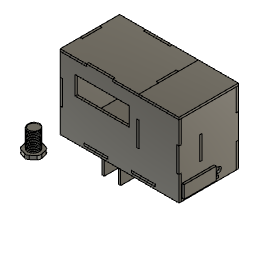
Tetrabytes (Autodesk Fusion 360 design; units mm, degrees)
Autodesk Fusion 360 part; units mm, degrees
note: some values were not read from the file. Chosen so that the rebuilt part matches the saved one: which face or edge a step refers to; which bodies a step acts on; where a thread starts. Set by a fixed rule: which sketch regions a step uses.
(part 1 of 2)
sketch "Sketch1" plane through (0, 0, 0) normal (0, 1, 0) x (1, 0, 0) in component "Front"
  line L0 (0, 0) -> (160, 0)
  line L1 (160, 0) -> (160, -100)
  line L2 (160, -100) -> (0, -100)
  line L3 (0, -100) -> (0, 0)
  line L4 (3, 0) -> (3, -100) construction
  line L5 (0, -3) -> (160, -3) construction
  line L6 (160, -6) -> (0, -6) construction
  line L7 (32, -3) -> (64, -3)
  line L8 (64, -3) -> (64, -6)
  line L9 (64, -6) -> (32, -6)
  line L10 (32, -6) -> (32, -3)
  line L11 (96, -3) -> (128, -3)
  line L12 (128, -3) -> (128, -6)
  line L13 (128, -6) -> (96, -6)
  line L14 (96, -6) -> (96, -3)
  line L15 (0, -66.6667) -> (3, -66.6667)
  line L16 (3, -66.6667) -> (3, -33.3333)
  line L17 (3, -33.3333) -> (0, -33.3333)
  line L18 (0, -33.3333) -> (0, -66.6667)
  line L19 (80, -100) -> (80, -87.8783) construction
  line L20 (157, -66.6667) -> (157, -33.3333)
  line L21 (160, -66.6667) -> (157, -66.6667)
  line L22 (157, -33.3333) -> (160, -33.3333)
  line L23 (160, -33.3333) -> (160, -66.6667)
  line L24 (157, 0) -> (157, -100) construction
  dimension "d1" = 160
  dimension "d8" = 100
  dimension "d9" = 3
  dimension "d10" = 3
  dimension "d11" = 3
  dimension "d12" = 32
  dimension "d13" = 32
  dimension "d14" = 32
  dimension "d15" = 32
  dimension "d16" = 33.3333
  dimension "d17" = 33.3333
  constraint horizontal L0
  constraint vertical L1
  constraint horizontal L2
  constraint vertical L3
  constraint coincident L0.start L3.end
  constraint coincident L0 L4.start
  constraint coincident L2 L4.end
  constraint perpendicular L2 L4
  constraint coincident L3 L5.start
  constraint coincident L1 L5.end
  constraint coincident L1 L6.start
  constraint coincident L3 L6.end
  constraint perpendicular L3 L6
  constraint horizontal L5
  constraint horizontal L7
  constraint vertical L8
  constraint horizontal L9
  constraint vertical L10
  constraint coincident L6 L8.end
  constraint coincident L5 L7.start
  constraint horizontal L11
  constraint vertical L12
  constraint horizontal L13
  constraint vertical L14
  constraint coincident L6 L12.end
  constraint coincident L5 L11.start
  constraint horizontal L15
  constraint vertical L16
  constraint horizontal L17
  constraint vertical L18
  constraint coincident L4 L16.end
  constraint coincident L3 L15.start
  constraint midpoint L2 L19.start
  constraint perpendicular L2 L19
  constraint symmetric L4.start L19 L24.start
  constraint symmetric L4.end L19 L24.end
  constraint symmetric L15.start L19 L21.start
  constraint symmetric L15.end L19 L20.start
  constraint symmetric L16.end L19 L20.end
  constraint symmetric L17.end L19 L22.end
  measures "d1" distance of L0.start L0.end
  measures "d8" distance of L0.start L2.end
  measures "d9" distance of L0 L5
  measures "d10" distance of L5 L6
  measures "d11" distance of L3 L4
  measures "d12" distance of L3 L10
  measures "d13" distance of L8 L10
  measures "d14" distance of L8 L14
  measures "d15" distance of L12 L14
  measures "d16" distance of L4.start L17
  measures "d17" distance of L15 L17
extrude "Extrude1" add sketch "Sketch1" along normal blind 3 contours L0 L1 L2 L3 L15 L16 L17 L20 L21 L22 makes body 1 in component "Front"
sketch "Sketch1 (2)" plane through (157, 0, 0) normal (1, 0, 0) x (0, 1, 0) in component "right"
  line L0 (0, 66.6667) -> (0, 33.3333)
  line L1 (0, 33.3333) -> (3, 33.3333)
  line L2 (3, 33.3333) -> (3, 66.6667)
  line L3 (3, 66.6667) -> (0, 66.6667)
  line L4 (0, 0) -> (80, 0)
  line L5 (80, 0) -> (80, 100)
  line L6 (80, 100) -> (0, 100)
  line L7 (0, 100) -> (0, 0)
  line L8 (0, 0) -> (3, 0)
  line L9 (0, 0) -> (0, 33.3333)
  line L10 (0, 100) -> (3, 100)
  line L11 (80, 3) -> (0, 3) construction
  line L12 (0, 6) -> (80, 6) construction
  line L13 (77, 0) -> (77, 100) construction
  line L14 (26.6667, 3) -> (53.3333, 3)
  line L15 (53.3333, 3) -> (53.3333, 6)
  line L16 (53.3333, 6) -> (26.6667, 6)
  line L17 (26.6667, 6) -> (26.6667, 3)
  line L18 (77, 66.6667) -> (80, 66.6667)
  line L19 (80, 66.6667) -> (80, 33.3333)
  line L20 (80, 33.3333) -> (77, 33.3333)
  line L21 (77, 33.3333) -> (77, 66.6667)
  line L22 (40, 100) -> (40, 92.4464) construction
  line L23 (0, 33.3333) -> (3, 33.3333)
  line L24 (3, 0) -> (3, 100) construction
  line L25 (3, 66.6667) -> (0, 66.6667)
  line L26 (0, 66.6667) -> (0, 33.3333)
  line L27 (3, 33.3333) -> (3, 66.6667)
  dimension "d20" = 80
  dimension "d21" = 3
  dimension "d22" = 3
  dimension "d23" = 3
  dimension "d24" = 26.6667
  dimension "d25" = 26.6667
  dimension "d26" = 33.3333
  dimension "d27" = 33.3333
  constraint horizontal L4
  constraint vertical L5
  constraint horizontal L6
  constraint vertical L7
  constraint collinear L4 L8
  constraint collinear L7 L9
  constraint collinear L6 L10
  constraint coincident L5 L11.start
  constraint coincident L9 L11.end
  constraint coincident L9 L12.start
  constraint coincident L5 L12.end
  constraint perpendicular L5 L12
  constraint coincident L4 L13.start
  constraint coincident L6 L13.end
  constraint perpendicular L6 L13
  constraint horizontal L11
  constraint horizontal L14
  constraint vertical L15
  constraint horizontal L16
  constraint vertical L17
  constraint coincident L12 L15.end
  constraint coincident L11 L14.start
  constraint horizontal L18
  constraint vertical L19
  constraint horizontal L20
  constraint vertical L21
  constraint coincident L5 L19.end
  constraint coincident L13 L18.start
  constraint midpoint L6 L22.start
  constraint perpendicular L6 L22
  constraint symmetric L13.start L22 L8.end
  constraint symmetric L13.end L22 L10.end
  constraint symmetric L18.start L22 L2.end
  constraint symmetric L18.end L22 L0.start
  constraint symmetric L19.end L22 L0.end
  constraint symmetric L20.end L22 L1.end
  measures "d20" distance of L4.start L4.end
  measures "d21" distance of L4 L11
  measures "d22" distance of L11 L12
  measures "d23" distance of L5 L13
  measures "d24" distance of L5 L15
  measures "d25" distance of L15 L17
  measures "d26" distance of L4 L20
  measures "d27" distance of L18 L20
extrude "Extrude1'" add sketch "Sketch1 (2)" along normal blind 3 separate body makes body 2 in component "right"
ref_plane "WorkPlane1" through (80, 40, 50) normal (1, 0, 0) x (0, 0, -1)
ref_plane "WorkPlane2" through (80, 40, 50) normal (0, -1, 0) x (-1, 0, 0)
mirror "MirrorComponent1" about plane through (0, 0, 0) normal (0, 0, 1) of bodies 1 makes body 3 in component "Front(Mirror)"
mirror "MirrorComponent2" about plane through (0, 0, 0) normal (0, 0, 1) of bodies 2 makes body 4 in component "right(Mirror)"
combine "Combine1" operation cut target body 2 tool bodies 1 3 body 3 seen with x (1, 0, 0) y (0, -1, 0) z (0, 0, -1) at (0, 80, 0) keep tools in component "right"
combine "Combine1'" operation cut target body 4 tool bodies 3 1 body 3 seen with x (-1, 0, 0) y (0, -1, 0) z (0, 0, 1) at (160, 80, 0) body 1 seen with x (-1, 0, 0) y (0, 1, 0) z (0, 0, -1) at (160, 0, 0) keep tools in component "right(Mirror)"
sketch "Sketch1 (3)" plane through (0, 0, 6) normal (0, 0, -1) x (1, 0, 0) in component "base"
  line L0 (64, 0) -> (32, 0)
  line L1 (32, 0) -> (32, -3)
  line L2 (32, -3) -> (64, -3)
  line L3 (64, -3) -> (64, 0)
  line L4 (0, -80) -> (160, -80)
  line L5 (160, -80) -> (160, 0)
  line L6 (160, 0) -> (0, 0)
  line L7 (0, 0) -> (0, -80)
  line L8 (0, -3) -> (0, -77)
  line L9 (0, 0) -> (160, 0)
  line L10 (160, -3) -> (160, -77)
  line L11 (0, -80) -> (160, -80)
  constraint horizontal L4
  constraint vertical L5
  constraint horizontal L6
  constraint vertical L7
  constraint collinear L7 L8
  constraint collinear L6 L9
  constraint collinear L5 L10
  constraint collinear L4 L11
extrude "Extrude1''" add sketch "Sketch1 (3)" along normal blind 3 separate body makes body 5 in component "base"
combine "Combine1''" operation cut target body 5 tool bodies 1 keep tools in component "base"
combine "Combine2" operation cut target body 5 tool bodies 2 keep tools in component "base"
combine "Combine3" operation cut target body 5 tool bodies 3 body 3 seen with x (1, 0, 0) y (0, -1, 0) z (0, 0, -1) at (0, 80, 0) keep tools in component "base"
combine "Combine4" operation cut target body 5 tool bodies 4 body 4 seen with x (-1, 0, 0) y (0, 1, 0) z (0, 0, -1) at (160, 0, 0) keep tools in component "base"
ref_plane "WorkPlane3" through (103, 40, 50) normal (1, 0, 0) x (0, -1, 0)
sketch "Sketch1 (4)" plane through (103, 40, 50) normal (1, 0, 0) x (0, 1, 0) in component "divider"
  line L0 (-40, 50) -> (40, 50)
  line L1 (40, 50) -> (40, -47)
  line L2 (40, -47) -> (-40, -47)
  line L3 (-40, -47) -> (-40, 50)
  line L4 (37, 50) -> (-37, 50)
  line L5 (40, 16.6667) -> (40, 50)
  line L6 (-40, 16.6667) -> (-40, 50)
  line L7 (37, -47) -> (13.3333, -47) construction
  line L8 (-40, -44) -> (40, -44)
  line L9 (-37, 50) -> (-37, -47)
  line L10 (-13.3333, -47) -> (13.3333, -47)
  line L11 (13.3333, -47) -> (13.3333, -44)
  line L12 (13.3333, -44) -> (-13.3333, -44)
  line L13 (-13.3333, -44) -> (-13.3333, -47)
  line L14 (-40, 19.6667) -> (-37, 19.6667)
  line L15 (-37, 19.6667) -> (-37, -13.6667)
  line L16 (-37, -13.6667) -> (-40, -13.6667)
  line L17 (-40, -13.6667) -> (-40, 19.6667)
  line L18 (0, 50) -> (0, 36.6243) construction
  line L19 (40, -13.6667) -> (40, 19.6667)
  line L20 (37, 50) -> (37, -47)
  line L21 (37, 19.6667) -> (37, -13.6667)
  line L22 (37, -13.6667) -> (40, -13.6667)
  line L23 (40, 19.6667) -> (37, 19.6667)
  dimension "d33" = 3
  dimension "d34" = 3
  dimension "d35" = 26.6667
  dimension "d36" = 26.6667
  dimension "d37" = 33.3333
  dimension "d38" = 33.3333
  constraint horizontal L0
  constraint vertical L1
  constraint horizontal L2
  constraint vertical L3
  constraint collinear L0 L4
  constraint collinear L1 L5
  constraint collinear L3 L6
  constraint collinear L2 L7
  constraint coincident L3 L8.start
  constraint coincident L1 L8.end
  constraint coincident L4 L9.start
  constraint coincident L2 L9.end
  constraint perpendicular L8 L9
  constraint vertical L9
  constraint horizontal L10
  constraint vertical L11
  constraint horizontal L12
  constraint vertical L13
  constraint coincident L8 L11.end
  constraint coincident L2 L10.start
  constraint horizontal L14
  constraint vertical L15
  constraint horizontal L16
  constraint vertical L17
  constraint coincident L9 L15.end
  constraint coincident L3 L14.start
  constraint midpoint L4 L18.start
  constraint perpendicular L4 L18
  constraint symmetric L4.end L18 L4.start
  constraint symmetric L9.end L18 L7.start
  constraint symmetric L14.start L18 L19.end
  constraint symmetric L14.end L18 L21.start
  constraint symmetric L15.end L18 L21.end
  constraint symmetric L16.end L18 L19.start
  measures "d33" distance of L2 L8
  measures "d34" distance of L3 L9
  measures "d35" distance of L3 L13
  measures "d36" distance of L11 L13
  measures "d37" distance of L2 L16
  measures "d38" distance of L14 L16
extrude "Extrude1'''" add sketch "Sketch1 (4)" along normal blind 3 separate body contours L0 L4 L8 L9 L12 L15 L20 L21 | L3 L6 L9 L14 L15 L16 L17 | L1 L5 L19 L20 L21 L22 L23 | L2 L8 L10 L11 L12 L13 makes body 6 in component "divider"
combine "Combine1'''" operation cut target body 1 tool bodies 6 keep tools in component "Front"
combine "Combine1''''" operation cut target body 3 tool bodies 6 body 6 seen with x (1, 0, 0) y (0, -1, 0) z (0, 0, -1) at (0, 80, 0) keep tools in component "Front(Mirror)"
combine "Combine5" operation cut target body 5 tool bodies 6 keep tools in component "base"
sketch "Sketch2" plane through (106, 0, 0) normal (1, 0, 0) x (0, 1, 0) in component "divider"
  line L0 (77, 36.3333) -> (80, 36.3333)
  line L1 (80, 36.3333) -> (80, 69.6667)
  line L2 (80, 69.6667) -> (77, 69.6667)
  line L3 (77, 69.6667) -> (77, 100)
  line L4 (77, 100) -> (3, 100)
  line L5 (3, 100) -> (3, 69.6667)
  line L6 (3, 69.6667) -> (0, 69.6667)
  line L7 (0, 69.6667) -> (0, 36.3333)
  line L8 (0, 36.3333) -> (3, 36.3333)
  line L9 (3, 36.3333) -> (3, 6)
  line L10 (3, 6) -> (26.6667, 6)
  line L11 (26.6667, 6) -> (26.6667, 3)
  line L12 (26.6667, 3) -> (53.3333, 3)
  line L13 (53.3333, 3) -> (53.3333, 6)
  line L14 (53.3333, 6) -> (77, 6)
  line L15 (77, 6) -> (77, 36.3333)
  line L16 (77, 6) -> (62, 6)
  line L17 (62, 6) -> (62, 21)
  line L18 (62, 21) -> (77, 21)
  line L19 (77, 21) -> (77, 6)
  dimension "d41" = 15
  dimension "d42" = 15
  constraint horizontal L16
  constraint vertical L17
  constraint horizontal L18
  constraint vertical L19
  constraint collinear L14 L16
  constraint collinear L15 L19
  measures "d41" distance of L14.end L18.end
  measures "d42" distance of L17.end L18.end
extrude "Extrude2" cut sketch "Sketch2" against normal up to surface (3 mm away) contours L14 L15 L16 L17 L18 L19 bodies 6 in component "divider"
sketch "Sketch1 (5)" plane through (0, 0, 100) normal (0, 0, 1) x (-1, 0, 0) in component "electronics cover"
  line L0 (-160, -80) -> (0, -80)
  line L1 (0, -80) -> (0, -77)
  line L2 (0, -77) -> (-160, -77)
  line L3 (-160, -77) -> (-160, -80)
  line L4 (0, -80) -> (-106, -80)
  line L5 (-106, -80) -> (-106, 0)
  line L6 (-106, 0) -> (0, 0)
  line L7 (0, 0) -> (0, -80)
  line L8 (0, -26.6667) -> (0, -53.3333)
  line L9 (-32, 0) -> (-64, 0)
  line L10 (-103, -77) -> (-103, -3)
  line L11 (-3, 0) -> (-3, -80) construction
  line L12 (0, -3) -> (-106, -3) construction
  line L13 (-35.3333, 0) -> (-70.6667, 0)
  line L14 (-70.6667, 0) -> (-70.6667, -3)
  line L15 (-70.6667, -3) -> (-35.3333, -3)
  line L16 (-35.3333, -3) -> (-35.3333, 0)
  line L17 (0, -26.6667) -> (-3, -26.6667)
  line L18 (-3, -26.6667) -> (-3, -53.3333)
  line L19 (-3, -53.3333) -> (0, -53.3333)
  line L20 (0, -53.3333) -> (0, -26.6667)
  line L21 (-53, -80) -> (-53, -70.5557) construction
  line L22 (-106, -40) -> (-94.7877, -40) construction
  line L23 (-106, -26.6667) -> (-103, -26.6667)
  line L24 (-103, -26.6667) -> (-103, -53.3333)
  line L25 (-106, -26.6667) -> (-106, -53.3333)
  line L26 (-106, -53.3333) -> (-106, -26.6667)
  line L27 (-103, 0) -> (-103, -80) construction
  line L28 (-103, -53.3333) -> (-106, -53.3333)
  line L29 (-35.3333, -77) -> (-35.3333, -80)
  line L30 (-70.6667, -77) -> (-35.3333, -77)
  line L31 (-32, -80) -> (-64, -80)
  line L32 (-70.6667, -80) -> (-70.6667, -77)
  line L33 (0, -77) -> (-106, -77) construction
  line L34 (-35.3333, -80) -> (-70.6667, -80)
  line L35 (-106, -77) -> (-106, -3)
  dimension "d45" = 3
  dimension "d46" = 3
  dimension "d47" = 35.3333
  dimension "d48" = 35.3333
  dimension "d49" = 26.6667
  dimension "d50" = 26.6667
  constraint horizontal L4
  constraint vertical L5
  constraint horizontal L6
  constraint vertical L7
  constraint collinear L0 L4
  constraint collinear L7 L8
  constraint collinear L6 L9
  constraint coincident L6 L11.start
  constraint coincident L4 L11.end
  constraint coincident L7 L12.start
  constraint coincident L5 L12.end
  constraint vertical L11
  constraint horizontal L12
  constraint horizontal L13
  constraint vertical L14
  constraint horizontal L15
  constraint vertical L16
  constraint coincident L12 L14.end
  constraint coincident L6 L13.start
  constraint horizontal L17
  constraint vertical L18
  constraint horizontal L19
  constraint vertical L20
  constraint coincident L11 L18.end
  constraint coincident L7 L8.start
  constraint midpoint L4 L21.start
  constraint perpendicular L2 L21
  constraint midpoint L5 L22.start
  constraint perpendicular L5 L22
  constraint symmetric L8.start L21 L23.start
  constraint symmetric L8.end L21 L25.end
  constraint symmetric L11.start L21 L27.start
  constraint symmetric L11.end L21 L27.end
  constraint symmetric L17.end L21 L23.end
  constraint symmetric L18.end L21 L24.end
  constraint symmetric L9.start L22 L31.start
  constraint symmetric L9.end L22 L31.end
  constraint symmetric L12.start L22 L1.end
  constraint symmetric L12.end L22 L33.end
  constraint symmetric L13.start L22 L29.end
  constraint symmetric L13.end L22 L32.start
  constraint symmetric L14.end L22 L30.start
  constraint symmetric L15.end L22 L29.start
  constraint collinear L5 L35
  measures "d45" distance of L6 L12
  measures "d46" distance of L7 L11
  measures "d47" distance of L5 L14
  measures "d48" distance of L14 L16
  measures "d49" distance of L6 L17
  measures "d50" distance of L17 L19
extrude "Extrude1''''" add sketch "Sketch1 (5)" against normal blind 3 separate body contours L0 L2 L4 L5 L32 | L2 L5 L10 L28 L35 | L2 L5 L6 L7 L9 L10 L14 L15 L16 L17 L18 L19 L23 L24 L30 L35 | L0 L1 L2 L4 L7 L29 L31 makes body 7 in component "electronics cover"
combine "Combine2'" operation cut target body 1 tool bodies 7 keep tools in component "Front"
combine "Combine2''" operation cut target body 4 tool bodies 7 body 7 seen with x (-1, 0, 0) y (0, 1, 0) z (0, 0, -1) at (160, 0, 0) keep tools in component "right(Mirror)"
combine "Combine2'''" operation cut target body 3 tool bodies 7 body 7 seen with x (1, 0, 0) y (0, -1, 0) z (0, 0, -1) at (0, 80, 0) keep tools in component "Front(Mirror)"
combine "Combine1'''''" operation cut target body 6 tool bodies 7 keep tools in component "divider"
sketch "Sketch1 (6)" plane through (0, 0, 100) normal (0, 0, 1) x (-1, 0, 0) in component "Food cover"
  line L0 (-106, -80) -> (-106, -77)
  line L1 (-106, -77) -> (-160, -77)
  line L2 (-160, -77) -> (-160, -80)
  line L3 (-160, -80) -> (-106, -80)
  line L4 (-106, -80) -> (-160, -80)
  line L5 (-160, -80) -> (-160, 0)
  line L6 (-160, 0) -> (-106, 0)
  line L7 (-106, 0) -> (-106, -80)
  line L8 (-160, 0) -> (-157, 0)
  line L9 (-160, -77) -> (-160, -3)
  line L10 (-103, -3) -> (-103, -26.6667)
  line L11 (-106, -77) -> (-106, -53.3333)
  constraint horizontal L4
  constraint vertical L5
  constraint horizontal L6
  constraint vertical L7
  constraint collinear L3 L4
  constraint collinear L6 L8
  constraint collinear L5 L9
  constraint collinear L7 L11
extrude "Extrude1'''''" add sketch "Sketch1 (6)" against normal blind 3 separate body makes body 8 in component "Food cover"
combine "Combine3'" operation cut target body 1 tool bodies 8 keep tools in component "Front"
combine "Combine2''''" operation cut target body 2 tool bodies 8 keep tools in component "right"
combine "Combine3''" operation cut target body 3 tool bodies 8 body 8 seen with x (1, 0, 0) y (0, -1, 0) z (0, 0, -1) at (0, 80, 0) keep tools in component "Front(Mirror)"
sketch "Sketch1 (7)" plane through (157, 0, 0) normal (-1, 0, 0) x (0, -1, 0) in component "hopper"
  line L0 (-3, 97) -> (-77, 97)
  line L1 (-77, 97) -> (-77, 66.6667)
  line L2 (-77, 66.6667) -> (-80, 66.6667)
  line L3 (-80, 66.6667) -> (-80, 33.3333)
  line L4 (-80, 33.3333) -> (-77, 33.3333)
  line L5 (-77, 33.3333) -> (-77, 0)
  line L6 (-77, 0) -> (-3, 0)
  line L7 (-3, 0) -> (-3, 33.3333)
  line L8 (-3, 33.3333) -> (0, 33.3333)
  line L9 (0, 33.3333) -> (0, 66.6667)
  line L10 (0, 66.6667) -> (-3, 66.6667)
  line L11 (-3, 66.6667) -> (-3, 97)
  line L12 (-26.6667, 6) -> (-26.6667, 3)
  line L13 (-26.6667, 3) -> (-53.3333, 3)
  line L14 (-53.3333, 3) -> (-53.3333, 6)
  line L15 (-53.3333, 6) -> (-26.6667, 6)
  line L16 (-28, 16) -> (-3, 16)
  line L17 (-3, 16) -> (-3, 6)
  line L18 (-3, 6) -> (-28, 6)
  line L19 (-28, 6) -> (-28, 16)
  line L20 (-26.6667, 6) -> (-3, 6)
  dimension "d55" = 25
  dimension "d56" = 10
  constraint horizontal L16
  constraint vertical L17
  constraint horizontal L18
  constraint vertical L19
  constraint collinear L7 L17
  constraint collinear L18 L20
  measures "d55" distance of L16.start L16.end
  measures "d56" distance of L16.start L18.end
ref_plane "WorkPlane4" through (104.5, 69.5, 31) normal (0, 0, -1) x (0, -1, 0)
ref_plane "WorkPlane5" through (80, 40, 23.25) normal (0, 0, 1) x (-1, 0, 0)
sketch "Sketch2 (2)" plane through (80, 40, 23.25) normal (0, 0, 1) x (1, 0, 0) in component "hopper"
  line L0 (77, -37) -> (26, -37)
  line L1 (26, -37) -> (26, -12)
  line L2 (26, -12) -> (77, -12)
  line L3 (77, -12) -> (77, -37)
  line L4 (77, -37) -> (77, 37)
  line L5 (48, -37) -> (77, -37)
  line L6 (26, -13.3333) -> (26, -37)
  line L7 (77, -37) -> (77, 37)
  line L8 (26, -40) -> (26, 40)
  dimension "d59" = 25
  constraint horizontal L0
  constraint vertical L1
  constraint horizontal L2
  constraint vertical L3
  constraint collinear L3 L4
  constraint collinear L0 L5
  constraint collinear L1 L8
  measures "d59" distance of L0 L2
sketch "Sketch3" plane through (104.5, 69.5, 31) normal (0, 0, -1) x (1, 0, 0) in component "hopper"
  line L0 (52.5, 66.5) -> (1.5, 66.5)
  line L1 (1.5, 66.5) -> (1.5, -7.5)
  line L2 (1.5, -7.5) -> (52.5, -7.5)
  line L3 (52.5, -7.5) -> (52.5, 66.5)
  line L4 (52.5, -7.5) -> (23.5, -7.5)
  line L5 (52.5, 66.5) -> (52.5, -7.5)
  line L6 (52.5, 66.5) -> (1.5, 66.5)
  line L7 (1.5, 16.1667) -> (1.5, 42.8333)
  constraint horizontal L0
  constraint vertical L1
  constraint horizontal L2
  constraint vertical L3
  constraint collinear L2 L4
  constraint collinear L3 L5
  constraint collinear L0 L6
  constraint collinear L1 L7
loft "Loft1" add profiles "Sketch2 (2)", "Sketch1 (7)" section 1 section 2 contours L7 L15 L16 L17 L18 L19 L20 separate body makes body 9 in component "hopper"
shell "Shell1" thickness 1 removed faces 1 at (123, 19.6667, 23.25) on bodies 9 in component "hopper"
sketch "Sketch4" plane through (0, 0, 6) normal (0, 0, 1) x (-1, 0, 0) in component "hopper"
  line L0 (-103, -53.3333) -> (-106, -53.3333)
  line L1 (-106, -53.3333) -> (-106, -26.6667)
  line L2 (-106, -26.6667) -> (-103, -26.6667)
  line L3 (-103, -26.6667) -> (-103, -53.3333)
  line L4 (-3, -26.6667) -> (-3, -3)
  line L5 (-3, -3) -> (-32, -3)
  line L6 (-32, -3) -> (-32, 0)
  line L7 (-32, 0) -> (-64, 0)
  line L8 (-64, 0) -> (-64, -3)
  line L9 (-64, -3) -> (-96, -3)
  line L10 (-96, -3) -> (-96, 0)
  line L11 (-96, 0) -> (-128, 0)
  line L12 (-128, 0) -> (-128, -3)
  line L13 (-128, -3) -> (-157, -3)
  line L14 (-157, -3) -> (-157, -26.6667)
  line L15 (-157, -26.6667) -> (-160, -26.6667)
  line L16 (-160, -26.6667) -> (-160, -53.3333)
  line L17 (-160, -53.3333) -> (-157, -53.3333)
  line L18 (-157, -53.3333) -> (-157, -77)
  line L19 (-157, -77) -> (-128, -77)
  line L20 (-128, -77) -> (-128, -80)
  line L21 (-128, -80) -> (-96, -80)
  line L22 (-96, -80) -> (-96, -77)
  line L23 (-96, -77) -> (-64, -77)
  line L24 (-64, -77) -> (-64, -80)
  line L25 (-64, -80) -> (-32, -80)
  line L26 (-32, -80) -> (-32, -77)
  line L27 (-32, -77) -> (-3, -77)
  line L28 (-3, -77) -> (-3, -53.3333)
  line L29 (-3, -53.3333) -> (0, -53.3333)
  line L30 (0, -53.3333) -> (0, -26.6667)
  line L31 (0, -26.6667) -> (-3, -26.6667)
  line L32 (-157, -3) -> (-106, -3)
  line L33 (-106, -3) -> (-106, -28)
  line L34 (-106, -28) -> (-157, -28)
  line L35 (-157, -28) -> (-157, -3)
  line L36 (-106, -26.6667) -> (-106, -3)
  line L37 (-157, -3) -> (-157, -77)
  line L38 (-157, -28) -> (-106, -28)
  constraint horizontal L32
  constraint vertical L33
  constraint horizontal L34
  constraint vertical L35
  constraint collinear L13 L32
  constraint collinear L33 L36
  constraint collinear L35 L37
  constraint collinear L34 L38
extrude "Extrude1''''''" add sketch "Sketch4" along normal up to near side of body 9 contours L1 L13 L14 L32 L33 L34 L35 L36 L37 L38 bodies 9 in component "hopper"
sketch "Sketch5" plane through (157, 0, 0) normal (1, 0, 0) x (0, 1, 0) in component "hopper"
  line L0 (28, 23.25) -> (3, 23.25)
  line L1 (3, 6) -> (28, 6)
  line L2 (28, 6) -> (28, 23.25)
  line L3 (3, 23.25) -> (3, 6)
  line L4 (4, 7.3939) -> (27, 7.3939)
  line L5 (27, 7.3939) -> (27, 17.3939)
  line L6 (27, 17.3939) -> (4, 17.3939)
  line L7 (4, 17.3939) -> (4, 7.3939)
  line L8 (3, 23.25) -> (28, 23.25)
  line L9 (28, 23.25) -> (28, 6)
  line L10 (28, 6) -> (3, 6)
  line L11 (3, 6) -> (3, 23.25)
  line L12 (27, 23.25) -> (4, 23.25)
  line L13 (4, 23.25) -> (4, 7.3939)
  line L14 (4, 7.3939) -> (27, 7.3939)
  line L15 (27, 7.3939) -> (27, 23.25)
  dimension "d108" = 10
  constraint horizontal L4
  constraint vertical L5
  constraint horizontal L6
  constraint vertical L7
  constraint collinear L4 L14
  constraint collinear L7 L13
  constraint collinear L5 L15
  measures "d108" distance of L4.end L5.end
extrude "Extrude2'" cut sketch "Sketch5" against normal up to surface (1 mm away) contours L4 L5 L6 L7 L13 L14 L15 bodies 9 in component "hopper"
sketch "Sketch2 (3)" plane through (160, 0, 0) normal (1, 0, 0) x (0, 1, 0) in component "right"
  line L0 (77, 97) -> (3, 97)
  line L1 (3, 97) -> (3, 66.6667)
  line L2 (3, 66.6667) -> (0, 66.6667)
  line L3 (0, 66.6667) -> (0, 33.3333)
  line L4 (0, 33.3333) -> (3, 33.3333)
  line L5 (3, 33.3333) -> (3, 0)
  line L6 (3, 0) -> (77, 0)
  line L7 (77, 0) -> (77, 33.3333)
  line L8 (77, 33.3333) -> (80, 33.3333)
  line L9 (80, 33.3333) -> (80, 66.6667)
  line L10 (80, 66.6667) -> (77, 66.6667)
  line L11 (77, 66.6667) -> (77, 97)
  line L12 (26.6667, 3) -> (26.6667, 6)
  line L13 (26.6667, 6) -> (53.3333, 6)
  line L14 (53.3333, 6) -> (53.3333, 3)
  line L15 (53.3333, 3) -> (26.6667, 3)
  line L16 (4, 17.3939) -> (27, 17.3939)
  line L17 (27, 17.3939) -> (27, 7.3939)
  line L18 (27, 7.3939) -> (4, 7.3939)
  line L19 (4, 7.3939) -> (4, 17.3939)
  line L20 (27, 23.25) -> (4, 23.25)
  line L21 (4, 23.25) -> (4, 7.3939)
  line L22 (4, 7.3939) -> (27, 7.3939)
  line L23 (27, 7.3939) -> (27, 23.25)
  dimension "d109" = 10
  constraint horizontal L16
  constraint vertical L17
  constraint horizontal L18
  constraint vertical L19
  constraint collinear L17 L23
  constraint collinear L18 L22
  constraint collinear L19 L21
  measures "d109" distance of L16.end L17.end
extrude "Extrude2''" cut sketch "Sketch2 (3)" against normal up to surface (3 mm away) contours L16 L17 L18 L19 L21 L22 L23 bodies 2 in component "right"
sketch "Sketch3 (2)" plane through (160, 0, 0) normal (1, 0, 0) x (0, 1, 0) in component "right"
  line L0 (77, 97) -> (3, 97)
  line L1 (3, 97) -> (3, 66.6667)
  line L2 (3, 66.6667) -> (0, 66.6667)
  line L3 (0, 66.6667) -> (0, 33.3333)
  line L4 (0, 33.3333) -> (3, 33.3333)
  line L5 (3, 33.3333) -> (3, 0)
  line L6 (3, 0) -> (77, 0)
  line L7 (77, 0) -> (77, 33.3333)
  line L8 (77, 33.3333) -> (80, 33.3333)
  line L9 (80, 33.3333) -> (80, 66.6667)
  line L10 (80, 66.6667) -> (77, 66.6667)
  line L11 (77, 66.6667) -> (77, 97)
  line L12 (26.6667, 3) -> (26.6667, 6)
  line L13 (26.6667, 6) -> (53.3333, 6)
  line L14 (53.3333, 6) -> (53.3333, 3)
  line L15 (53.3333, 3) -> (26.6667, 3)
  arc A0 (52.2036, 8.5572) -> (52.2005, 15.6972) centre (53.35, 12.1277) ccw
  arc A1 (52.2005, 15.6972) -> (52.2036, 8.5572) centre (47.225, 12.125) ccw
  line L16 (4, 17.3939) -> (27, 17.3939)
  line L17 (27, 17.3939) -> (27, 7.3939)
  line L18 (27, 7.3939) -> (4, 7.3939)
  line L19 (4, 7.3939) -> (4, 17.3939)
  dimension "d71" = 12.25
  dimension "d73" = 7.5
  dimension "d74" = 29.775
  constraint coincident A0.centre A1
  constraint tangent L13 A1
  measures "d71" diameter of A1
  measures "d73" diameter of A0
  measures "d74" distance of L7 A1.centre
extrude "Extrude3" cut sketch "Sketch3 (2)" against normal up to surface (3 mm away) contours A0 A1 bodies 2 in component "right"
sketch "Sketch2 (4)" plane through (0, 0, 0) normal (0, -1, 0) x (1, 0, 0) in component "Front"
  line L0 (32, 6) -> (64, 6)
  line L1 (64, 6) -> (64, 3)
  line L2 (64, 3) -> (32, 3)
  line L3 (32, 3) -> (32, 6)
  line L4 (96, 6) -> (128, 6)
  line L5 (128, 6) -> (128, 3)
  line L6 (128, 3) -> (96, 3)
  line L7 (96, 3) -> (96, 6)
  line L8 (103, 69.6667) -> (106, 69.6667)
  line L9 (106, 69.6667) -> (106, 36.3333)
  line L10 (106, 36.3333) -> (103, 36.3333)
  line L11 (103, 36.3333) -> (103, 69.6667)
  line L12 (160, 97) -> (70.6667, 97)
  line L13 (70.6667, 97) -> (70.6667, 100)
  line L14 (70.6667, 100) -> (35.3333, 100)
  line L15 (35.3333, 100) -> (35.3333, 97)
  line L16 (35.3333, 97) -> (0, 97)
  line L17 (0, 97) -> (0, 66.6667)
  line L18 (0, 66.6667) -> (3, 66.6667)
  line L19 (3, 66.6667) -> (3, 33.3333)
  line L20 (3, 33.3333) -> (0, 33.3333)
  line L21 (0, 33.3333) -> (0, 0)
  line L22 (0, 0) -> (160, 0)
  line L23 (160, 0) -> (160, 33.3333)
  line L24 (160, 33.3333) -> (157, 33.3333)
  line L25 (157, 33.3333) -> (157, 66.6667)
  line L26 (157, 66.6667) -> (160, 66.6667)
  line L27 (160, 66.6667) -> (160, 97)
  line L28 (20, 55) -> (93, 55)
  line L29 (93, 55) -> (93, 80)
  line L30 (93, 80) -> (20, 80)
  line L31 (20, 80) -> (20, 55)
  dimension "d77" = 73
  dimension "d78" = 25
  dimension "d80" = 20
  dimension "d81" = 10
  constraint horizontal L28
  constraint vertical L29
  constraint horizontal L30
  constraint vertical L31
  measures "d77" distance of L29 L31
  measures "d78" distance of L28 L30
  measures "d80" distance of L14 L30
  measures "d81" distance of L11 L29
extrude "Extrude2'''" cut sketch "Sketch2 (4)" against normal up to surface (3 mm away) contours L28 L29 L30 L31 bodies 1 in component "Front"
sketch "Sketch1 (8)" plane through (160, 0, 0) normal (1, 0, 0) x (0, 1, 0) in component "hatch door"
  line L0 (26.6667, 3) -> (26.6667, 6)
  line L1 (26.6667, 6) -> (47.225, 6)
  arc A0 (52.2005, 15.6972) -> (47.225, 6) centre (47.225, 12.125) ccw
  arc A1 (52.2036, 8.5572) -> (52.2005, 15.6972) centre (53.35, 12.1277) ccw
  arc A2 (47.225, 6) -> (52.2036, 8.5572) centre (47.225, 12.125) ccw
  line L2 (47.225, 6) -> (53.3333, 6)
  line L3 (53.3333, 6) -> (53.3333, 3)
  line L4 (53.3333, 3) -> (26.6667, 3)
  line L5 (77, 97) -> (3, 97)
  line L6 (3, 97) -> (3, 66.6667)
  line L7 (3, 66.6667) -> (0, 66.6667)
  line L8 (0, 66.6667) -> (0, 33.3333)
  line L9 (0, 33.3333) -> (3, 33.3333)
  line L10 (3, 33.3333) -> (3, 0)
  line L11 (3, 0) -> (77, 0)
  line L12 (77, 0) -> (77, 33.3333)
  line L13 (77, 33.3333) -> (80, 33.3333)
  line L14 (80, 33.3333) -> (80, 66.6667)
  line L15 (80, 66.6667) -> (77, 66.6667)
  line L16 (77, 66.6667) -> (77, 97)
  line L17 (4, 3.946) -> (47.225, 3.946)
  line L18 (47.225, 3.946) -> (47.225, 20.946)
  line L19 (47.225, 20.946) -> (4, 20.946)
  line L20 (4, 20.946) -> (4, 3.946)
  line L21 (4, 17.3939) -> (27, 17.3939)
  line L22 (27, 17.3939) -> (27, 7.3939)
  line L23 (27, 7.3939) -> (4, 7.3939)
  line L24 (4, 7.3939) -> (4, 17.3939)
  constraint horizontal L17
  constraint vertical L18
  constraint horizontal L19
  constraint vertical L20
  constraint coincident A0.centre L18
extrude "Extrude1'''''''" add sketch "Sketch1 (8)" along normal blind 3 separate body contours L0 L1 A0 L17 L18 L19 L20 L21 L22 L23 | L0 L1 L17 L18 | A0 L18 | L20 L21 L22 L23 L24 makes body 10 in component "hatch door"
sketch "Sketch1 (9)" plane through (0, 0, 3) normal (0, 0, -1) x (1, 0, 0) in component "mount"
  line L0 (103, -26.6667) -> (106, -26.6667)
  line L1 (106, -26.6667) -> (106, -53.3333)
  line L2 (106, -53.3333) -> (103, -53.3333)
  line L3 (103, -53.3333) -> (103, -26.6667)
  line L4 (3, -53.3333) -> (3, -77)
  line L5 (3, -77) -> (32, -77)
  line L6 (32, -77) -> (32, -80)
  line L7 (32, -80) -> (64, -80)
  line L8 (64, -80) -> (64, -77)
  line L9 (64, -77) -> (96, -77)
  line L10 (96, -77) -> (96, -80)
  line L11 (96, -80) -> (128, -80)
  line L12 (128, -80) -> (128, -77)
  line L13 (128, -77) -> (157, -77)
  line L14 (157, -77) -> (157, -53.3333)
  line L15 (157, -53.3333) -> (160, -53.3333)
  line L16 (160, -53.3333) -> (160, -26.6667)
  line L17 (160, -26.6667) -> (157, -26.6667)
  line L18 (157, -26.6667) -> (157, -3)
  line L19 (157, -3) -> (128, -3)
  line L20 (128, -3) -> (128, 0)
  line L21 (128, 0) -> (96, 0)
  line L22 (96, 0) -> (96, -3)
  line L23 (96, -3) -> (64, -3)
  line L24 (64, -3) -> (64, 0)
  line L25 (64, 0) -> (32, 0)
  line L26 (32, 0) -> (32, -3)
  line L27 (32, -3) -> (3, -3)
  line L28 (3, -3) -> (3, -26.6667)
  line L29 (3, -26.6667) -> (0, -26.6667)
  line L30 (0, -26.6667) -> (0, -53.3333)
  line L31 (0, -53.3333) -> (3, -53.3333)
  line L32 (53.3333, -77) -> (78.3333, -77)
  line L33 (78.3333, -77) -> (78.3333, -3)
  line L34 (78.3333, -3) -> (53.3333, -3)
  line L35 (53.3333, -3) -> (53.3333, -77)
  line L36 (160, -3) -> (0, -3)
  line L37 (160, -77) -> (0, -77)
  line L38 (0, -3) -> (0, -77)
  dimension "d87" = 53.3333
  dimension "d88" = 25
  constraint horizontal L32
  constraint vertical L33
  constraint horizontal L34
  constraint vertical L35
  constraint collinear L34 L36
  constraint collinear L32 L37
  measures "d87" distance of L35 L38
  measures "d88" distance of L33 L35
extrude "Extrude1''''''''" add sketch "Sketch1 (9)" along normal blind 3 separate body contours L9 L23 L32 L33 L34 L35 L36 L37 makes body 11 in component "mount"
sketch "Sketch2 (5)" plane through (78.3333, 0, 0) normal (1, 0, 0) x (0, 1, 0) in component "mount"
  line L0 (77, 3) -> (3, 3)
  line L1 (3, 3) -> (3, 0)
  line L2 (3, 0) -> (77, 0)
  line L3 (77, 0) -> (77, 3)
  line L4 (3, -22) -> (77, -22)
  line L5 (77, -22) -> (77, 3)
  line L6 (77, 3) -> (3, 3)
  line L7 (3, 3) -> (3, -22)
  dimension "d91" = 25
  constraint horizontal L4
  constraint vertical L5
  constraint horizontal L6
  constraint vertical L7
  constraint collinear L0 L6
  constraint collinear L1 L7
  constraint collinear L3 L5
  measures "d91" distance of L4 L6
extrude "Extrude2''''" add sketch "Sketch2 (5)" against normal blind 3 contours L2 L4 L5 L7 bodies 11 in component "mount"
sketch "Sketch3 (3)" plane through (53.3333, 0, 0) normal (-1, 0, 0) x (0, -1, 0) in component "mount"
  line L0 (-3, 3) -> (-77, 3)
  line L1 (-77, 3) -> (-77, 0)
  line L2 (-77, 0) -> (-3, 0)
  line L3 (-3, 0) -> (-3, 3)
  line L4 (-77, 3) -> (-3, 3)
  line L5 (-3, 3) -> (-3, -22)
  line L6 (-3, -22) -> (-77, -22)
  line L7 (-77, -22) -> (-77, 3)
  line L8 (-3, -22) -> (-3, 0)
  line L9 (-77, -22) -> (-3, -22)
  constraint horizontal L4
  constraint vertical L5
  constraint horizontal L6
  constraint vertical L7
  constraint coincident L0.end L1.start
  constraint collinear L5 L8
  constraint collinear L6 L9
extrude "Extrude3'" add sketch "Sketch3 (3)" against normal blind 3 contours L2 L5 L6 L7 L8 L9 bodies 11 in component "mount"
sketch "Sketch1 (10)" plane through (0, 0, 0) normal (0, -1, 0) x (1, 0, 0)
  line L0 (20, 80) -> (93, 80)
  line L1 (93, 80) -> (93, 55)
  line L2 (93, 55) -> (20, 55)
  line L3 (20, 55) -> (20, 80)
  line L4 (32, 6) -> (64, 6)
  line L5 (64, 6) -> (64, 3)
  line L6 (64, 3) -> (32, 3)
  line L7 (32, 3) -> (32, 6)
  line L8 (96, 6) -> (128, 6)
  line L9 (128, 6) -> (128, 3)
  line L10 (128, 3) -> (96, 3)
  line L11 (96, 3) -> (96, 6)
  line L12 (103, 69.6667) -> (106, 69.6667)
  line L13 (106, 69.6667) -> (106, 36.3333)
  line L14 (106, 36.3333) -> (103, 36.3333)
  line L15 (103, 36.3333) -> (103, 69.6667)
  line L16 (160, 97) -> (70.6667, 97)
  line L17 (70.6667, 97) -> (70.6667, 100)
  line L18 (70.6667, 100) -> (35.3333, 100)
  line L19 (35.3333, 100) -> (35.3333, 97)
  line L20 (35.3333, 97) -> (0, 97)
  line L21 (0, 97) -> (0, 66.6667)
  line L22 (0, 66.6667) -> (3, 66.6667)
  line L23 (3, 66.6667) -> (3, 33.3333)
  line L24 (3, 33.3333) -> (0, 33.3333)
  line L25 (0, 33.3333) -> (0, 0)
  line L26 (0, 0) -> (160, 0)
  line L27 (160, 0) -> (160, 33.3333)
  line L28 (160, 33.3333) -> (157, 33.3333)
  line L29 (157, 33.3333) -> (157, 66.6667)
  line L30 (157, 66.6667) -> (160, 66.6667)
  line L31 (160, 66.6667) -> (160, 97)
sketch "Sketch2 (6)" plane through (160, 0, 0) normal (1, 0, 0) x (0, 1, 0)
  line L0 (26.6667, 3) -> (26.6667, 6)
  line L1 (26.6667, 6) -> (47.225, 6)
  arc A0 (52.2005, 15.6972) -> (47.225, 6) centre (47.225, 12.125) ccw
  arc A1 (52.2036, 8.5572) -> (52.2005, 15.6972) centre (53.35, 12.1277) ccw
  arc A2 (47.225, 6) -> (52.2036, 8.5572) centre (47.225, 12.125) ccw
  line L2 (47.225, 6) -> (53.3333, 6)
  line L3 (53.3333, 6) -> (53.3333, 3)
  line L4 (53.3333, 3) -> (26.6667, 3)
  line L5 (77, 97) -> (3, 97)
  line L6 (3, 97) -> (3, 66.6667)
  line L7 (3, 66.6667) -> (0, 66.6667)
  line L8 (0, 66.6667) -> (0, 33.3333)
  line L9 (0, 33.3333) -> (3, 33.3333)
  line L10 (3, 33.3333) -> (3, 0)
  line L11 (3, 0) -> (77, 0)
  line L12 (77, 0) -> (77, 33.3333)
  line L13 (77, 33.3333) -> (80, 33.3333)
  line L14 (80, 33.3333) -> (80, 66.6667)
  line L15 (80, 66.6667) -> (77, 66.6667)
  line L16 (77, 66.6667) -> (77, 97)
  line L17 (4, 17.3939) -> (27, 17.3939)
  line L18 (27, 17.3939) -> (27, 7.3939)
  line L19 (27, 7.3939) -> (4, 7.3939)
  line L20 (4, 7.3939) -> (4, 17.3939)
sketch "Sketch3 (4)" plane through (0, 0, 0) normal (-1, 0, 0) x (0, -1, 0)
  line L0 (-53.3333, 97) -> (-77, 97)
  line L1 (-77, 97) -> (-77, 66.6667)
  line L2 (-77, 66.6667) -> (-80, 66.6667)
  line L3 (-80, 66.6667) -> (-80, 33.3333)
  line L4 (-80, 33.3333) -> (-77, 33.3333)
  line L5 (-77, 33.3333) -> (-77, 0)
  line L6 (-77, 0) -> (-3, 0)
  line L7 (-3, 0) -> (-3, 33.3333)
  line L8 (-3, 33.3333) -> (0, 33.3333)
  line L9 (0, 33.3333) -> (0, 66.6667)
  line L10 (0, 66.6667) -> (-3, 66.6667)
  line L11 (-3, 66.6667) -> (-3, 97)
  line L12 (-3, 97) -> (-26.6667, 97)
  line L13 (-26.6667, 97) -> (-26.6667, 100)
  line L14 (-26.6667, 100) -> (-53.3333, 100)
  line L15 (-53.3333, 100) -> (-53.3333, 97)
  line L16 (-26.6667, 6) -> (-26.6667, 3)
  line L17 (-26.6667, 3) -> (-53.3333, 3)
  line L18 (-53.3333, 3) -> (-53.3333, 6)
  line L19 (-53.3333, 6) -> (-26.6667, 6)
sketch "Sketch4 (2)" plane through (0, 80, 0) normal (0, 1, 0) x (-1, 0, 0)
  line L0 (-70.6667, 97) -> (-160, 97)
  line L1 (-160, 97) -> (-160, 66.6667)
  line L2 (-160, 66.6667) -> (-157, 66.6667)
  line L3 (-157, 66.6667) -> (-157, 33.3333)
  line L4 (-157, 33.3333) -> (-160, 33.3333)
  line L5 (-160, 33.3333) -> (-160, 0)
  line L6 (-160, 0) -> (0, 0)
  line L7 (0, 0) -> (0, 33.3333)
  line L8 (0, 33.3333) -> (-3, 33.3333)
  line L9 (-3, 33.3333) -> (-3, 66.6667)
  line L10 (-3, 66.6667) -> (0, 66.6667)
  line L11 (0, 66.6667) -> (0, 97)
  line L12 (0, 97) -> (-35.3333, 97)
  line L13 (-35.3333, 97) -> (-35.3333, 100)
  line L14 (-35.3333, 100) -> (-70.6667, 100)
  line L15 (-70.6667, 100) -> (-70.6667, 97)
  line L16 (-64, 6) -> (-32, 6)
  line L17 (-32, 6) -> (-32, 3)
  line L18 (-32, 3) -> (-64, 3)
  line L19 (-64, 3) -> (-64, 6)
  line L20 (-128, 6) -> (-96, 6)
  line L21 (-96, 6) -> (-96, 3)
  line L22 (-96, 3) -> (-128, 3)
  line L23 (-128, 3) -> (-128, 6)
  line L24 (-103, 36.3333) -> (-106, 36.3333)
  line L25 (-106, 36.3333) -> (-106, 69.6667)
  line L26 (-106, 69.6667) -> (-103, 69.6667)
  line L27 (-103, 69.6667) -> (-103, 36.3333)
sketch "Sketch5 (2)" plane through (0, 0, 3) normal (0, 0, -1) x (1, 0, 0)
  line L0 (103, -26.6667) -> (106, -26.6667)
  line L1 (106, -26.6667) -> (106, -53.3333)
  line L2 (106, -53.3333) -> (103, -53.3333)
  line L3 (103, -53.3333) -> (103, -26.6667)
  line L4 (3, -53.3333) -> (3, -77)
  line L5 (3, -77) -> (32, -77)
  line L6 (32, -77) -> (32, -80)
  line L7 (32, -80) -> (64, -80)
  line L8 (64, -80) -> (64, -77)
  line L9 (64, -77) -> (96, -77)
  line L10 (96, -77) -> (96, -80)
  line L11 (96, -80) -> (128, -80)
  line L12 (128, -80) -> (128, -77)
  line L13 (128, -77) -> (157, -77)
  line L14 (157, -77) -> (157, -53.3333)
  line L15 (157, -53.3333) -> (160, -53.3333)
  line L16 (160, -53.3333) -> (160, -26.6667)
  line L17 (160, -26.6667) -> (157, -26.6667)
  line L18 (157, -26.6667) -> (157, -3)
  line L19 (157, -3) -> (128, -3)
  line L20 (128, -3) -> (128, 0)
  line L21 (128, 0) -> (96, 0)
  line L22 (96, 0) -> (96, -3)
  line L23 (96, -3) -> (64, -3)
  line L24 (64, -3) -> (64, 0)
  line L25 (64, 0) -> (32, 0)
  line L26 (32, 0) -> (32, -3)
  line L27 (32, -3) -> (3, -3)
  line L28 (3, -3) -> (3, -26.6667)
  line L29 (3, -26.6667) -> (0, -26.6667)
  line L30 (0, -26.6667) -> (0, -53.3333)
  line L31 (0, -53.3333) -> (3, -53.3333)
sketch "Sketch6" plane through (0, 0, 100) normal (0, 0, 1) x (-1, 0, 0)
  line L0 (-70.6667, -80) -> (-70.6667, -77)
  line L1 (-70.6667, -77) -> (-35.3333, -77)
  line L2 (-35.3333, -77) -> (-35.3333, -80)
  line L3 (-35.3333, -80) -> (0, -80)
  line L4 (0, -80) -> (0, -53.3333)
  line L5 (0, -53.3333) -> (-3, -53.3333)
  line L6 (-3, -53.3333) -> (-3, -26.6667)
  line L7 (-3, -26.6667) -> (0, -26.6667)
  line L8 (0, -26.6667) -> (0, 0)
  line L9 (0, 0) -> (-35.3333, 0)
  line L10 (-35.3333, 0) -> (-35.3333, -3)
  line L11 (-35.3333, -3) -> (-70.6667, -3)
  line L12 (-70.6667, -3) -> (-70.6667, 0)
  line L13 (-70.6667, 0) -> (-106, 0)
  line L14 (-106, 0) -> (-106, -26.6667)
  line L15 (-106, -26.6667) -> (-103, -26.6667)
  line L16 (-103, -26.6667) -> (-103, -53.3333)
  line L17 (-103, -53.3333) -> (-106, -53.3333)
  line L18 (-106, -53.3333) -> (-106, -80)
  line L19 (-106, -80) -> (-70.6667, -80)
sketch "Sketch7" plane through (0, 0, 100) normal (0, 0, 1) x (-1, 0, 0)
  line L0 (-106, -80) -> (-106, 0)
  line L1 (-106, 0) -> (-160, 0)
  line L2 (-160, 0) -> (-160, -80)
  line L3 (-160, -80) -> (-106, -80)
sketch "Sketch10" plane through (106, 0, 0) normal (1, 0, 0) x (0, 1, 0)
  line L0 (77, 97) -> (53.3333, 97)
  line L1 (53.3333, 97) -> (53.3333, 100)
  line L2 (53.3333, 100) -> (26.6667, 100)
  line L3 (26.6667, 100) -> (26.6667, 97)
  line L4 (26.6667, 97) -> (3, 97)
  line L5 (3, 97) -> (3, 69.6667)
  line L6 (3, 69.6667) -> (0, 69.6667)
  line L7 (0, 69.6667) -> (0, 36.3333)
  line L8 (0, 36.3333) -> (3, 36.3333)
  line L9 (3, 36.3333) -> (3, 6)
  line L10 (3, 6) -> (26.6667, 6)
  line L11 (26.6667, 6) -> (26.6667, 3)
  line L12 (26.6667, 3) -> (53.3333, 3)
  line L13 (53.3333, 3) -> (53.3333, 6)
  line L14 (53.3333, 6) -> (62, 6)
  line L15 (62, 6) -> (62, 21)
  line L16 (62, 21) -> (77, 21)
  line L17 (77, 21) -> (77, 36.3333)
  line L18 (77, 36.3333) -> (80, 36.3333)
  line L19 (80, 36.3333) -> (80, 69.6667)
  line L20 (80, 69.6667) -> (77, 69.6667)
  line L21 (77, 69.6667) -> (77, 97)
sketch "Sketch11" plane through (163, 0, 0) normal (1, 0, 0) x (0, 1, 0)
  line L0 (4, 20.946) -> (4, 3.946)
  line L1 (4, 3.946) -> (47.225, 3.946)
  line L2 (47.225, 3.946) -> (47.225, 20.946)
  line L3 (47.225, 20.946) -> (4, 20.946)
sketch "Sketch1 (11)" plane through (0, 28, 0) normal (0, 1, 0) x (-1, 0, 0) in component "divider2"
  line L0 (-103, 3) -> (-160, 3)
  line L1 (-160, 3) -> (-160, 97)
  line L2 (-160, 97) -> (-103, 97)
  line L3 (-103, 97) -> (-103, 3)
  line L4 (-96, 3) -> (-128, 3)
  line L5 (-160, 33.3333) -> (-160, 66.6667)
  line L6 (-103, 36.3333) -> (-103, 69.6667)
  line L7 (-70.6667, 97) -> (-160, 97)
  line L8 (-157, 97) -> (-157, 3)
  line L9 (-160, 6) -> (-103, 6)
  line L10 (-157, 34.3333) -> (-160, 34.3333)
  line L11 (-160, 34.3333) -> (-160, 65.6667)
  line L12 (-160, 65.6667) -> (-157, 65.6667)
  line L13 (-157, 65.6667) -> (-157, 34.3333)
  line L14 (-141, 3) -> (-122, 3)
  line L15 (-122, 3) -> (-122, 6)
  line L16 (-122, 6) -> (-141, 6)
  line L17 (-141, 6) -> (-141, 3)
  line L18 (-103, 21) -> (-103, 6)
  line L19 (-160, 0) -> (-160, 33.3333)
  line L20 (-128, 3) -> (-157, 3)
  line L21 (-157, 3) -> (-160, 3)
  line L22 (-131.5, 97) -> (-131.5, 90.1924) construction
  line L23 (-103, 65.6667) -> (-106, 65.6667)
  line L24 (-106, 34.3333) -> (-103, 34.3333)
  line L25 (-106, 65.6667) -> (-106, 34.3333)
  line L26 (-103, 33.3333) -> (-103, 66.6667)
  line L27 (-103, 34.3333) -> (-103, 65.6667)
  line L28 (-106, 97) -> (-106, 3)
  point P0 (-103, 33.3333)
  dimension "d121" = 3
  dimension "d122" = 3
  dimension "d123" = 57
  dimension "d124" = 94
  dimension "d125" = 19
  dimension "d126" = 19
  dimension "d127" = 31.3333
  dimension "d128" = 31.3333
  constraint horizontal L0
  constraint vertical L1
  constraint horizontal L2
  constraint vertical L3
  constraint collinear L0 L4
  constraint collinear L1 L5
  constraint collinear L3 L6
  constraint collinear L2 L7
  constraint coincident L2 L8.start
  constraint coincident L0 L8.end
  constraint perpendicular L0 L8
  constraint coincident L1 L9.start
  constraint coincident L3 L9.end
  constraint perpendicular L3 L9
  constraint horizontal L10
  constraint vertical L11
  constraint horizontal L12
  constraint vertical L13
  constraint coincident L5 L11.end
  constraint coincident L8 L10.start
  constraint horizontal L14
  constraint vertical L15
  constraint horizontal L16
  constraint vertical L17
  constraint coincident L9 L15.end
  constraint coincident L0 L14.start
  constraint midpoint L2 L22.start
  constraint perpendicular L2 L22
  constraint symmetric L5.start L22 P0
  constraint symmetric L5.end L22 L26.end
  constraint symmetric L8.start L22 L28.start
  constraint symmetric L8.end L22 L28.end
  constraint symmetric L10.start L22 L24.start
  constraint symmetric L10.end L22 L24.end
  constraint symmetric L11.end L22 L23.start
  constraint symmetric L12.end L22 L23.end
  measures "d121" distance of L5 L8
  measures "d122" distance of L4 L9
  measures "d123" distance of L18 L19
  measures "d124" distance of L7 L20
  measures "d125" distance of L17 L19
  measures "d126" distance of L15 L17
  measures "d127" distance of L10 L21
  measures "d128" distance of L10 L12
extrude "Extrude1'''''''''" add sketch "Sketch1 (11)" along normal blind 3 separate body contours L0 L4 L9 L14 L15 L16 L17 L20 | L2 L7 L8 L9 L13 L16 L25 L28 | L3 L6 L23 L24 L25 L26 L27 L28 | L1 L5 L8 L10 L11 L12 L13 makes body 12 in component "divider2"
combine "Combine6" operation cut target body 5 tool bodies 12 keep tools in component "base"
combine "Combine2'''''" operation cut target body 6 tool bodies 12 keep tools in component "divider"
combine "Combine3'''" operation cut target body 2 tool bodies 12 keep tools in component "right"
sketch "Sketch12" plane through (0, 31, 0) normal (0, 1, 0) x (-1, 0, 0)
  line L0 (-157, 97) -> (-157, 65.6667)
  line L1 (-157, 65.6667) -> (-160, 65.6667)
  line L2 (-160, 65.6667) -> (-160, 34.3333)
  line L3 (-160, 34.3333) -> (-157, 34.3333)
  line L4 (-157, 34.3333) -> (-157, 6)
  line L5 (-157, 6) -> (-141, 6)
  line L6 (-141, 6) -> (-141, 3)
  line L7 (-141, 3) -> (-122, 3)
  line L8 (-122, 3) -> (-122, 6)
  line L9 (-122, 6) -> (-106, 6)
  line L10 (-106, 6) -> (-106, 34.3333)
  line L11 (-106, 34.3333) -> (-103, 34.3333)
  line L12 (-103, 34.3333) -> (-103, 65.6667)
  line L13 (-103, 65.6667) -> (-106, 65.6667)
  line L14 (-106, 65.6667) -> (-106, 97)
  line L15 (-106, 97) -> (-157, 97)
sketch "Sketch3 (5)" plane through (0, 0, 0) normal (0, 0, 1) x (1, 0, 0) in component "bolt"
  circle A0 centre (3.3069, -39.2276) radius 8
  line L0 (13.0238, -30.1768) -> (0.3272, -26.2872)
  line L1 (0.3272, -26.2872) -> (-9.3897, -35.3379)
  line L2 (-9.3897, -35.3379) -> (-6.4099, -48.2783)
  line L3 (-6.4099, -48.2783) -> (6.2867, -52.168)
  line L4 (6.2867, -52.168) -> (16.0036, -43.1172)
  line L5 (16.0036, -43.1172) -> (13.0238, -30.1768)
  circle A1 centre (3.3069, -39.2276) radius 13.2791
  point P0 (3.3069, -39.2276)
  dimension "d151" = 16
  dimension "d152" = 11.5
  constraint coincident P0 A0.centre
  constraint coincident L0.start A1
  measures "d151" diameter of A0
  measures "d152" distance of P0 L5
extrude "Extrude3''" add sketch "Sketch3 (5)" along normal blind 5 separate body contours A0 | L0 L1 L2 L3 L4 L5 makes body 13 in component "bolt"
sketch "Sketch4 (3)" plane through (0, 0, 5) normal (0, 0, 1) x (-1, 0, 0) in component "bolt"
  line L0 (-16.0036, 43.1172) -> (-13.0238, 30.1768)
  line L1 (-13.0238, 30.1768) -> (-0.3272, 26.2872)
  line L2 (-0.3272, 26.2872) -> (9.3897, 35.3379)
  line L3 (9.3897, 35.3379) -> (6.4099, 48.2783)
  line L4 (6.4099, 48.2783) -> (-6.2867, 52.168)
  line L5 (-6.2867, 52.168) -> (-16.0036, 43.1172)
  line L6 (6.4099, 48.2783) -> (-13.0238, 30.1768) construction
  line L7 (-0.3272, 26.2872) -> (-6.2867, 52.168) construction
  line L8 (-16.0036, 43.1172) -> (9.3897, 35.3379) construction
  circle A0 centre (-3.3069, 39.2276) radius 8
  dimension "d157" = 16
  constraint coincident L3.end L4.start
  constraint coincident L0.end L1.start
  constraint coincident L1.end L2.start
  constraint coincident L4.end L5.start
  constraint coincident L0.start L5.end
  constraint coincident L2.end L3.start
  constraint midpoint L8 A0.centre
  measures "d157" diameter of A0
extrude "Extrude5" add sketch "Sketch4 (3)" along normal blind 25 contours A0 bodies 13 in component "bolt"
sketch "Sketch6 (2)" plane through (53.3333, 0, 0) normal (-1, 0, 0) x (0, -1, 0) in component "mount"
  line L0 (-3, 3) -> (-77, 3)
  line L1 (-77, 3) -> (-77, -22)
  line L2 (-77, -22) -> (-3, -22)
  line L3 (-3, -22) -> (-3, 3)
  circle A0 centre (-40, -9.5) radius 9.75
  dimension "d161" = 12.5
  dimension "d162" = 19.5
  dimension "d163" = 37
  measures "d161" distance of L2 A0.centre
  measures "d162" diameter of A0
  measures "d163" distance of L1 A0.centre
extrude "Extrude7" add sketch "Sketch6 (2)" along normal blind 3.5 contours A0 bodies 11 in component "mount"
hole "Hole7" at (49.8333, 40, -9.5) direction (1, 0, 0) diameter 14.023 depth 6.5 tip angle 118 bodies 11 in component "mount"